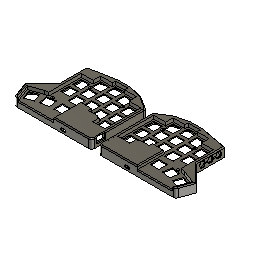
top_33332_3 (Autodesk Fusion 360 design; units mm, degrees)
Autodesk Fusion 360 part; units mm, degrees
sketch "case_plate_33332_3" plane through (0, 0, 0) normal (0, 0, 1) x (1, 0, 0)
  line L0 (67.6888, 46.482) -> (67.5953, 46.5)
  line L1 (28.1017, 41.4312) -> (8.5, 29.0512)
  line L2 (48.3769, 46.5) -> (28.1017, 41.4312)
  line L3 (8.5, -52.72) -> (126.2948, -52.72)
  line L4 (107.5, -5.3353) -> (107.5, 38.826)
  line L5 (8.5, 29.0512) -> (8.5, -52.72)
  line L6 (126.2948, -52.72) -> (133.9348, -31.7293)
  line L7 (67.5953, 46.5) -> (48.3769, 46.5)
  line L8 (107.5, 38.826) -> (67.6888, 46.482)
  line L9 (133.9348, -31.7293) -> (107.5, -5.3353)
  line L10 (110.5, -4.0913) -> (110.5, 41.3041)
  line L11 (67.8811, 49.5) -> (48.0076, 49.5)
  line L12 (128.3954, -55.72) -> (137.4081, -30.9579)
  line L13 (137.4081, -30.9579) -> (110.5, -4.0913)
  line L14 (5.5, -55.72) -> (128.3954, -55.72)
  line L15 (26.9069, 44.2248) -> (5.5, 30.7047)
  line L16 (48.0076, 49.5) -> (26.9069, 44.2248)
  line L17 (5.5, 30.7047) -> (5.5, -55.72)
  line L18 (110.5, 41.3041) -> (67.8811, 49.5)
  line L19 (108.7, 39.8172) -> (67.7096, 47.7)
  line L20 (135.3241, -31.4207) -> (108.7, -4.8377)
  line L21 (127.135, -53.92) -> (135.3241, -31.4207)
  line L22 (108.7, -4.8377) -> (108.7, 39.8172)
  line L23 (7.3, -53.92) -> (127.135, -53.92)
  line L24 (67.7096, 47.7) -> (48.2292, 47.7)
  line L25 (48.2292, 47.7) -> (27.6238, 42.5487)
  line L26 (7.3, 29.7126) -> (7.3, -53.92)
  line L27 (27.6238, 42.5487) -> (7.3, 29.7126)
  line L28 (109.3, -4.5889) -> (109.3, 40.3128)
  line L29 (6.7, -54.52) -> (127.5552, -54.52)
  line L30 (6.7, 30.0433) -> (6.7, -54.52)
  line L31 (109.3, 40.3128) -> (68.0288, 48.2496)
  line L32 (48.1553, 48.3) -> (27.3848, 43.1074)
  line L33 (27.3848, 43.1074) -> (6.7, 30.0433)
  line L34 (127.5552, -54.52) -> (136.0188, -31.2664)
  line L35 (67.7668, 48.3) -> (48.1553, 48.3)
  line L36 (68.0288, 48.2496) -> (67.7668, 48.3)
  line L37 (136.0188, -31.2664) -> (109.3, -4.5889)
  circle A0 centre (32, 20.5) radius 2.2
  circle A1 centre (84, 20.5) radius 2.2
  circle A2 centre (100.1356, -23.3241) radius 2.2
  line L38 (10.5, -31.61) -> (10.5, -49.61)
  line L39 (43.5, -31.61) -> (10.5, -31.61)
  line L40 (43.5, -49.61) -> (43.5, -31.61)
  line L41 (10.5, -49.61) -> (43.5, -49.61)
  line L42 (47.025, -46.99) -> (47.025, -52.84)
  line L43 (55.825, -52.84) -> (55.825, -46.99)
  line L44 (55.825, -46.99) -> (47.025, -46.99)
  line L45 (66.825, -47.975) -> (57.825, -47.975)
  line L46 (57.825, -47.975) -> (57.825, -51.475)
  line L47 (57.825, -51.475) -> (66.825, -51.475)
  line L48 (66.825, -51.475) -> (66.825, -47.975)
  line L49 (122.6064, -22.1718) -> (114.8282, -14.3936)
  line L50 (114.8282, -14.3936) -> (108.3936, -20.8282)
  line L51 (108.3936, -20.8282) -> (110.7259, -23.1606)
  line L52 (118.9049, -25.8732) -> (122.6064, -22.1718)
  line L53 (43.2, -28.45) -> (43.2, -19.55)
  line L54 (43.2, -19.55) -> (34.7125, -19.55)
  line L55 (34.6, -19.6909) -> (34.6, -28.45)
  line L56 (34.6, -28.45) -> (43.2, -28.45)
  line L57 (27, -13) -> (13, -13)
  line L58 (13, -13) -> (13, -27)
  line L59 (27, -27) -> (27, -13)
  line L60 (13, -27) -> (27, -27)
  line L61 (27, -8) -> (27, 6)
  line L62 (13, -8) -> (27, -8)
  line L63 (13, 6) -> (13, -8)
  line L64 (27, 6) -> (13, 6)
  line L65 (13, 25) -> (13, 11)
  line L66 (13, 11) -> (27, 11)
  line L67 (27, 25) -> (13, 25)
  line L68 (27, 11) -> (27, 25)
  line L69 (32, -15) -> (46, -15)
  line L70 (46, -1) -> (32, -1)
  line L71 (46, -15) -> (46, -1)
  line L72 (32, -1) -> (32, -15)
  line L73 (46, 4) -> (46, 18)
  line L74 (46, 18) -> (32, 18)
  line L75 (32, 4) -> (46, 4)
  line L76 (32, 18) -> (32, 4)
  line L77 (46, 37) -> (32, 37)
  line L78 (32, 23) -> (46, 23)
  line L79 (32, 37) -> (32, 23)
  line L80 (46, 23) -> (46, 37)
  line L81 (65, 4) -> (51, 4)
  line L82 (51, 4) -> (51, -10)
  line L83 (65, -10) -> (65, 4)
  line L84 (51, -10) -> (65, -10)
  line L85 (65, 23) -> (51, 23)
  line L86 (65, 9) -> (65, 23)
  line L87 (51, 23) -> (51, 9)
  line L88 (51, 9) -> (65, 9)
  line L89 (51, 42) -> (51, 28)
  line L90 (65, 28) -> (65, 42)
  line L91 (65, 42) -> (51, 42)
  line L92 (51, 28) -> (65, 28)
  line L93 (84, -1) -> (70, -1)
  line L94 (84, -15) -> (84, -1)
  line L95 (70, -15) -> (84, -15)
  line L96 (70, -1) -> (70, -15)
  line L97 (84, 4) -> (84, 18)
  line L98 (70, 18) -> (70, 4)
  line L99 (70, 4) -> (84, 4)
  line L100 (84, 18) -> (70, 18)
  line L101 (84, 23) -> (84, 37)
  line L102 (70, 23) -> (84, 23)
  line L103 (70, 37) -> (70, 23)
  line L104 (84, 37) -> (70, 37)
  line L105 (103, 6) -> (89, 6)
  line L106 (89, -8) -> (103, -8)
  line L107 (89, 6) -> (89, -8)
  line L108 (103, -8) -> (103, 6)
  line L109 (103, 11) -> (103, 25)
  line L110 (89, 25) -> (89, 11)
  line L111 (89, 11) -> (103, 11)
  line L112 (103, 25) -> (89, 25)
  line L113 (84, -23.8) -> (70, -23.8)
  line L114 (70, -37.8) -> (84, -37.8)
  line L115 (84, -37.8) -> (84, -23.8)
  line L116 (70, -23.8) -> (70, -37.8)
  line L117 (92.8078, -24.5706) -> (90.3767, -38.3579)
  line L118 (106.5951, -27.0017) -> (92.8078, -24.5706)
  line L119 (104.164, -40.789) -> (106.5951, -27.0017)
  line L120 (90.3767, -38.3579) -> (104.164, -40.789)
  line L121 (115.1353, -29.29) -> (110.347, -42.4457)
  line L122 (123.5027, -47.234) -> (128.291, -34.0783)
  line L123 (128.291, -34.0783) -> (115.1353, -29.29)
  line L124 (110.347, -42.4457) -> (123.5027, -47.234)
  line L125 (8.5, -29.75) -> (29.75, -29.75)
  line L126 (29.75, -29.75) -> (29.75, -19.7)
  line L127 (10.25, -29.75) -> (10.25, 27.75)
  line L128 (29.25, 27.75) -> (10.25, 27.75)
  line L129 (48.75, -17.75) -> (48.75, -12.75)
  line L130 (48.25, 39.75) -> (29.25, 39.75)
  line L131 (29.25, 39.75) -> (29.25, 27.75)
  line L132 (48.75, -12.75) -> (67.25, -12.75)
  line L133 (67.75, 39.75) -> (67.75, 44.75)
  line L134 (67.75, 44.75) -> (48.25, 44.75)
  line L135 (48.25, 44.75) -> (48.25, 39.75)
  line L136 (67.25, -55.72) -> (67.25, -12.75)
  line L137 (86.75, 27.75) -> (86.75, 39.75)
  line L138 (86.75, 39.75) -> (67.75, 39.75)
  line L139 (105.75, -24.0602) -> (105.75, -5.3353)
  line L140 (105.75, 27.75) -> (86.75, 27.75)
  line L141 (67.25, -40.55) -> (86.9722, -40.55)
  line L142 (86.9722, -40.55) -> (106.6135, -44.0133)
  line L143 (105.75, -24.0602) -> (111.608, -25.0931)
  line L144 (106.6135, -44.0133) -> (125.1463, -50.7587)
  line L145 (123.3406, -55.72) -> (131.8157, -32.4347)
  line L146 (111.7483, -25.1307) -> (133.4723, -33.0376)
  line L147 (107.5, -5.3353) -> (105.75, -5.3353)
  line L148 (32, -19.7) -> (29.75, -19.7)
  arc A3 (32, -19.7) -> (34.1857, -17.75) centre (32, -17.5) ccw
  line L149 (29.75, -17.75) -> (29.8143, -17.75)
  line L150 (34.1857, -17.75) -> (48.75, -17.75)
  line L151 (8.5, -30.95) -> (30.95, -30.95)
  line L152 (30.95, -30.95) -> (30.95, -20.9)
  line L153 (32, -20.9) -> (30.95, -20.9)
  arc A4 (32, -20.9) -> (35.0753, -18.95) centre (32, -17.5) ccw
  line L154 (35.0753, -18.95) -> (49.95, -18.95)
  line L155 (49.95, -18.95) -> (49.95, -13.95)
  line L156 (49.95, -13.95) -> (66.05, -13.95)
  line L157 (66.05, -55.72) -> (66.05, -13.95)
  line L158 (105.75, -5.3353) -> (105.75, 27.75)
  line L159 (111.608, -25.0931) -> (111.7483, -25.1307)
  line L160 (107.5, -22.5918) -> (107.5, -5.3353)
  line L161 (107.5, -22.5918) -> (111.9871, -23.383)
  line L162 (111.9871, -23.383) -> (112.275, -23.4601)
  line L163 (112.275, -23.4601) -> (133.327, -31.1224)
extrude "Extrude1" add sketch "case_plate_33332_3" against normal blind 7.6 contours L14 L29 L136 L145 | L10 L11 L12 L13 L14 L15 L16 L17 L18 L28 L29 L30 L31 L32 L33 L34 L35 L36 L37 L145 L157 | L14 L29 L136 L157 makes body 1
extrude "Extrude2" add sketch "case_plate_33332_3" against normal blind 6.8 contours L0 L1 L2 L3 L4 L5 L6 L7 L8 L9 L19 L20 L21 L22 L23 L24 L25 L26 L27 L145 L157 | L3 L23 L136 L145 | L3 L23 L136 L157 | L23 L29 L136 L145 | L19 L20 L21 L22 L23 L24 L25 L26 L27 L28 L29 L30 L31 L32 L33 L34 L35 L36 L37 L145 L157 | L23 L29 L136 L157 bodies 1
extrude "Extrude3" add sketch "case_plate_33332_3" along normal blind 1.6 contours L125 L126 L127 L128 L129 L130 L131 L132 L133 L134 L135 L136 L137 L138 L139 L140 L141 L142 L143 L144 L145 L146 L148 A3 L150 L158 L159 | L3 L23 L136 L145 | L3 L136 L141 L142 L144 L145 | L23 L29 L136 L145 | L14 L29 L136 L145 | A0 | A1 | A2 bodies 1
extrude "Extrude4" add sketch "case_plate_33332_3" along normal blind 7 contours L0 L1 L2 L4 L5 L7 L8 L125 L127 L128 L130 L131 L133 L134 L135 L137 L138 L140 L147 L158 | L0 L1 L2 L3 L4 L5 L6 L7 L8 L9 L19 L20 L21 L22 L23 L24 L25 L26 L27 L145 L157 | L6 L9 L139 L143 L146 L147 L159 L160 L161 L162 L163 | L3 L5 L45 L47 L48 L125 L126 L129 L132 L136 L148 A3 L150 L151 L152 L153 A4 L154 L155 L156 L157 | L3 L6 L145 L146 | L3 L23 L136 L157 | L19 L20 L21 L22 L23 L24 L25 L26 L27 L28 L29 L30 L31 L32 L33 L34 L35 L36 L37 L145 L157 | L23 L29 L136 L157 | L10 L11 L12 L13 L14 L15 L16 L17 L18 L28 L29 L30 L31 L32 L33 L34 L35 L36 L37 L145 L157 | L45 L47 L48 L157 | L14 L29 L136 L157 bodies 1
extrude "Extrude5" add sketch "case_plate_33332_3" along normal blind 1.6 from surface at 5.4 contours L9 L49 L50 L51 L52 L160 L161 L163 | L49 L50 L51 L52 L161 L162 L163 | L3 L5 L42 L43 L44 L45 L46 L47 L53 L54 L55 L56 L151 L152 L153 A4 L154 L155 L156 L157 | L3 L42 L43 L44 | L53 L54 L55 L56 A4 | L45 L46 L47 L157 | L38 L39 L40 L41 bodies 1
move_body "Move1" bodies 1 to x (1, 0, 0) y (0, 1, 0) z (0, 0, 1) at (0, 0, -1.6)
hole "Hole1" at (32, 20.5, 0) at (32, -17.5, 0) at (84, 20.5, 0) at (100.1356, -23.3241, 0) direction (0, 0, -1) diameter 2.4 depth 20 tip angle 180 countersink diameter 4.4 countersink angle 90 bodies 1
sketch "Sketch2" plane through (5.5, 0, 0) normal (-1, 0, 0) x (0, -1, 0)
  line L0 (-30.7047, 5.4) -> (-30.7047, -9.2)
  line L1 (-30.7047, -9.2) -> (55.72, -9.2)
  line L2 (55.72, -9.2) -> (55.72, 5.4)
  line L3 (55.72, 5.4) -> (-30.7047, 5.4)
  line L4 (-30.7047, -9.2) -> (55.72, -9.2)
  line L5 (55.72, 5.4) -> (-30.7047, 5.4)
  line L6 (55.72, -9.2) -> (55.72, 5.4)
  line L7 (-30.7047, 5.4) -> (-30.7047, -9.2)
  line L8 (49.61, 0) -> (31.61, 0) construction
  line L9 (27.8309, 4.2) -> (55.72, 4.2)
  line L10 (27.7335, -3.8) -> (55.72, -3.8)
  line L11 (34.61, 4.2) -> (34.61, -3.8)
  line L12 (46.61, 4.2) -> (46.61, -3.8)
extrude "Extrude6" cut sketch "Sketch2" against normal up to surface (3 mm away) contours L9 L10 L11 L12 bodies 1
chamfer "Chamfer1" distance 1 angle 45 4 edges at (5.5, -40.61, 4.2) (5.5, -34.61, 0.2) (5.5, -40.61, -3.8) (5.5, -46.61, 0.2) on bodies 1
sketch "cutout-pwr" plane through (0, -55.72, 0) normal (0, -1, 0) x (-1, 0, 0)
  line L0 (-128.3954, -5.4) -> (-113.5707, -5.4)
  line L1 (-75.8577, 0) -> (-75.8577, -5.4)
  line L2 (-113.5707, 0) -> (-75.8577, 0)
  line L3 (-113.5707, -5.4) -> (-113.5707, 0)
  line L4 (-5.5, 9.2) -> (-128.3954, 9.2)
  line L5 (-128.3954, 9.2) -> (-128.3954, -5.4)
  line L6 (-75.8577, -5.4) -> (-5.5, -5.4)
  line L7 (-5.5, -5.4) -> (-5.5, 9.2)
  line L8 (-55.825, 0) -> (-47.025, 0)
  line L9 (-53.425, 2.75) -> (-49.425, 2.75)
  line L10 (-49.425, 5.75) -> (-53.425, 5.75)
  arc A0 (-53.425, 5.75) -> (-53.425, 2.75) centre (-53.425, 4.25) ccw
  arc A1 (-49.425, 2.75) -> (-49.425, 5.75) centre (-49.425, 4.25) ccw
extrude "Extrude7" cut sketch "cutout-pwr" against normal up to surface (3 mm away) contours L9 L10 A0 A1 bodies 1
sketch "Sketch4" plane through (0, 0, -5.75) normal (0, 0, 1) x (-1, 0, 0)
  line L0 (-53.425, 52.72) -> (-49.425, 52.72)
  line L1 (-49.425, 52.72) -> (-49.425, 55.72)
  line L2 (-49.425, 55.72) -> (-53.425, 55.72)
  line L3 (-53.425, 55.72) -> (-53.425, 52.72)
  line L4 (-49.425, 54.22) -> (-53.425, 54.22)
  constraint midpoint L1 L4.start
  constraint midpoint L3 L4.end
extrude "Extrude8" cut sketch "Sketch4" against normal up to surface (2.65 mm away) contours L0 L1 L3 L4 bodies 1
chamfer "Chamfer2" distance 0.5 angle 45 4 edges at (51.425, -55.72, -2.75) (54.925, -55.72, -4.25) (51.425, -55.72, -5.75) (47.925, -55.72, -4.25) on bodies 1
sketch "magnet-8mm-long" plane through (110.5, 0, 0) normal (1, 0, 0) x (0, -1, 0)
  line L0 (-41.3041, -5.4) -> (4.0913, -5.4)
  line L1 (4.0913, 9.2) -> (-41.3041, 9.2)
  line L2 (-41.3041, 9.2) -> (-41.3041, -5.4)
  line L3 (4.0913, -5.4) -> (4.0913, 9.2)
  line L4 (-7.8821, 5.486) -> (-10.1962, 1.5222)
  line L5 (-10.1962, 1.5222) -> (-7.9205, -2.4639)
  line L6 (-1.0165, 1.4778) -> (-3.2922, 5.4639)
  line L7 (-3.3306, -2.486) -> (-1.0165, 1.4778)
  line L8 (-3.2922, 5.4639) -> (-7.8821, 5.486)
  line L9 (-7.9205, -2.4639) -> (-3.3306, -2.486)
  line L10 (-23.1962, 1.5222) -> (-20.9205, -2.4639)
  line L11 (-20.8821, 5.486) -> (-23.1962, 1.5222)
  line L12 (-16.3306, -2.486) -> (-14.0165, 1.4778)
  line L13 (-20.9205, -2.4639) -> (-16.3306, -2.486)
  line L14 (-16.2922, 5.4639) -> (-20.8821, 5.486)
  line L15 (-14.0165, 1.4778) -> (-16.2922, 5.4639)
  line L16 (-29.3306, -2.486) -> (-27.0165, 1.4778)
  line L17 (-33.9205, -2.4639) -> (-29.3306, -2.486)
  line L18 (-27.0165, 1.4778) -> (-29.2922, 5.4639)
  line L19 (-36.1962, 1.5222) -> (-33.9205, -2.4639)
  line L20 (-33.8821, 5.486) -> (-36.1962, 1.5222)
  line L21 (-29.2922, 5.4639) -> (-33.8821, 5.486)
  line L22 (-5.6064, 2.25) -> (-31.6064, 2.25)
  line L23 (-31.6064, 0.75) -> (-5.6064, 0.75)
  arc A0 (-31.6064, 2.25) -> (-31.6064, 0.75) centre (-31.6064, 1.5) ccw
  arc A1 (-5.6064, 0.75) -> (-5.6064, 2.25) centre (-5.6064, 1.5) ccw
  point P0 (-18.6064, 1.5)
  point P1 (-31.6064, 1.5)
  point P2 (-5.6064, 1.5)
  point P3 (-5.6064, 1.5)
  point P4 (-18.6064, 1.5)
  point P5 (-31.6064, 1.5)
extrude "Extrude9" cut sketch "magnet-8mm-long" against normal blind 2 contours L4 L5 L6 L7 L8 L9 L22 L23 A1 | L4 L5 L22 L23 A1 | L4 L5 L12 L15 L22 L23 | L11 L14 L15 L22 | L10 L11 L12 L15 L22 L23 | L10 L11 L16 L18 L22 L23 | L10 L12 L13 L23 | L16 L17 L18 L19 L20 L21 L22 L23 A0 | L16 L18 L22 L23 A0 bodies 1
sketch "magnet-8mm-short" plane through (53.1189, 53.2011, 0) normal (0.70656, 0.707653, 0) x (0.707653, -0.70656, 0)
  line L0 (100.4285, 5.5) -> (100.4285, 4.5)
  line L1 (93.4285, 5.5) -> (100.4285, 5.5)
  line L2 (93.4285, 4.5) -> (93.4285, 5.5)
  line L3 (100.4285, 4.5) -> (93.4285, 4.5)
  line L4 (81.0864, -5.4) -> (119.1108, -5.4)
  line L5 (119.1108, -5.4) -> (119.1108, 9.2)
  line L6 (119.1108, 9.2) -> (81.0864, 9.2)
  line L7 (81.0864, 9.2) -> (81.0864, -5.4)
  line L8 (111.7008, 1.4927) -> (109.4121, 5.4713)
  line L9 (102.5209, 1.5073) -> (104.8095, -2.4713)
  line L10 (104.8222, 5.4786) -> (102.5209, 1.5073)
  line L11 (109.4121, 5.4713) -> (104.8222, 5.4786)
  line L12 (104.8095, -2.4713) -> (109.3995, -2.4786)
  line L13 (109.3995, -2.4786) -> (111.7008, 1.4927)
  line L14 (91.3751, 5.4786) -> (86.7851, 5.4713)
  line L15 (93.6764, 1.5073) -> (91.3751, 5.4786)
  line L16 (84.4965, 1.4927) -> (86.7978, -2.4786)
  line L17 (86.7978, -2.4786) -> (91.3877, -2.4713)
  line L18 (86.7851, 5.4713) -> (84.4965, 1.4927)
  line L19 (91.3877, -2.4713) -> (93.6764, 1.5073)
  line L20 (107.1108, 2.25) -> (89.0864, 2.25)
  line L21 (89.0864, 0.75) -> (107.1108, 0.75)
  arc A0 (107.1108, 0.75) -> (107.1108, 2.25) centre (107.1108, 1.5) ccw
  arc A1 (89.0864, 2.25) -> (89.0864, 0.75) centre (89.0864, 1.5) ccw
  point P0 (107.1108, 1.5)
  point P1 (89.0864, 1.5)
  point P2 (107.1108, 1.5)
  point P3 (89.0864, 1.5)
extrude "Extrude10" cut sketch "magnet-8mm-short" against normal blind 2 contours L8 L9 L10 L11 L12 L13 L20 L21 A0 | L9 L10 L20 L21 A0 | L9 L10 L15 L19 L20 L21 | L14 L15 L16 L17 L18 L19 L20 L21 A1 | L15 L19 L20 L21 A1 bodies 1
extrude "Extrude11" cut sketch "magnet-8mm-short" against normal up to surface (3 mm away) contours L0 L1 L2 L3 bodies 1
chamfer "Chamfer3" distance 0.4 angle 45 30 edges at (131.3501, -24.9092, 0.493) (131.3545, -24.9137, -3.482) (128.9118, -22.4747, 2.475) (126.6321, -20.1985, 0.8607) (126.6347, -20.2011, -3.8643) (128.9207, -22.4836, -5.475) (118.4454, -12.0244, 0.8607) (118.4428, -12.0218, -3.8643) (116.1657, -9.7483, 2.475) (113.7274, -7.3138, 0.493) (113.7229, -7.3093, -3.482) (116.1568, -9.7393, -5.475) (110.5, 2.1735, 0.5041) (110.5, 2.1544, -3.4709) (110.5, 5.5872, -5.475) (110.5, 5.6256, 2.475) (110.5, 8.8379, 0.8569) (110.5, 8.8267, -3.868) (110.5, 15.386, 0.868) (110.5, 15.3748, -3.8569) (110.5, 18.5872, -5.475) (110.5, 18.6256, 2.475) (110.5, 21.8379, 0.8569) (110.5, 21.8267, -3.868) (110.5, 28.386, 0.868) (110.5, 31.6256, 2.475) (110.5, 28.3748, -3.8569) (110.5, 31.5872, -5.475) (110.5, 35.0584, 0.4709) (110.5, 35.0392, -3.5041) on bodies 1
fillet "Fillet1" radius 5 6 edges at (128.3954, -55.72, -1.9) (5.5, -55.72, -1.9) (5.5, 30.7047, -1.9) (26.9069, 44.2248, -1.9) (48.0076, 49.5, -1.9) (67.8811, 49.5, -1.9) on bodies 1
fillet "Fillet1" radius 5 6 edges at (6.7, 30.0433, -8.8) (27.3848, 43.1074, -8.8) (48.1553, 48.3, -8.8) (67.7668, 48.3, -8.8) (6.7, -54.52, -8.8) (127.5552, -54.52, -8.8) on bodies 1
fillet "Fillet1" radius 2 6 edges at (126.2948, -52.72, -5) (8.5, -52.72, -2.3) (8.5, 29.0512, -5) (28.1017, 41.4312, -5) (48.3769, 46.5, -5) (67.5953, 46.5, -5) on bodies 1
chamfer "Chamfer4" distance 1.5 angle 45 18 edges at (127.7623, -54.8157, 5.4) (133.5005, -41.694, 5.4) (124.1175, -55.72, 5.4) (127.5781, -44.0773, 5.4) (67.25, -34.235, 5.4) (38.875, -55.72, 5.4) (89.4245, 45.357, 5.4) (67.879, 49.4775, 5.4) (58.0139, 49.5, 5.4) (48.0122, 49.4625, 5.4) (37.548, 46.8851, 5.4) (26.9321, 44.166, 5.4) (17.0292, 37.9863, 5.4) (6.1211, 30.3624, 5.4) (5.5, -11.3856, 5.4) (6.9645, -54.2555, 5.4) (123.954, -17.5246, 5.4) (110.5, 18.6064, 5.4) on bodies 1
fillet "Fillet2" radius 1.5 1 edges at (95.2953, -55.72, 0) on bodies 1
mirror "Mirror1" about plane through (0, 0, 0) normal (1, 0, 0) of bodies 1 makes body 2
